Autodesk Inventor part; units mm, degrees
(part 2 of 2)
sketch "スケッチ18" plane through (0, 0, 0) normal (0, 0, 1) x (1, 0, 0)
  line L0 (54.4443, -3) -> (57.4443, -3)
  line L1 (57.4443, -3) -> (57.4443, -6)
  arc A0 (57.4443, -6) -> (59.4443, -6) centre (58.4443, -6) ccw
  line L2 (59.4443, -6) -> (64.4443, -6)
  arc A1 (64.4443, -6) -> (66.4443, -6) centre (65.4443, -6) ccw
  line L3 (66.4443, -6) -> (66.4443, -3)
  line L4 (66.4443, -3) -> (69.4443, -3)
  arc A2 (69.4443, -3) -> (71.4443, -3) centre (70.4443, -3) ccw
  line L5 (71.4443, -3) -> (82.8897, -3)
  arc A3 (82.8897, -3) -> (84.8897, -3) centre (83.8897, -3) ccw
  line L6 (84.8897, -3) -> (87.8897, -3)
  line L7 (87.8897, -3) -> (87.8897, -6)
  arc A4 (87.8897, -6) -> (89.8897, -6) centre (88.8897, -6) ccw
  line L8 (89.8897, -6) -> (94.8897, -6)
  arc A5 (94.8897, -6) -> (96.8897, -6) centre (95.8897, -6) ccw
  line L9 (96.8897, -6) -> (96.8897, -3)
  line L10 (96.8897, -3) -> (99.8897, -3)
  arc A6 (99.8897, -3) -> (101.8897, -3) centre (100.8897, -3) ccw
  line L11 (101.8897, -3) -> (104.885, -3)
  line L12 (104.885, -3) -> (104.885, -31.8586)
  arc A7 (104.885, -31.8586) -> (119.127, -45.896) centre (111.885, -39) ccw
  line L13 (119.127, -45.896) -> (127.6513, -45.7727)
  line L14 (127.6513, -45.7727) -> (121.0577, -50.8686)
  arc A8 (102.2194, -50.4706) -> (121.0577, -50.8686) centre (111.885, -39) ccw
  line L15 (102.2194, -50.4706) -> (49.4443, -6)
  line L16 (49.4443, -6) -> (49.4443, -3)
  line L17 (49.4443, -3) -> (52.4443, -3)
  arc A9 (52.4443, -3) -> (54.4443, -3) centre (53.4443, -3) ccw
  line L18 (99.1203, -14.609) -> (85.9579, -30.2295)
  arc A10 (85.9579, -30.2295) -> (86.0782, -31.6386) centre (86.7226, -30.8739) ccw
  line L19 (86.0782, -31.6386) -> (97.3043, -41.0982)
  arc A11 (97.3043, -41.0982) -> (98.9442, -40.2383) centre (97.9487, -40.3335) ccw
  arc A12 (100.7422, -32.304) -> (98.9442, -40.2383) centre (111.885, -39) ccw
  arc A13 (100.7422, -32.304) -> (100.885, -31.7889) centre (99.885, -31.7889) ccw
  line L20 (100.885, -31.7889) -> (100.885, -15.2534)
  arc A14 (100.885, -15.2534) -> (99.1203, -14.609) centre (99.885, -15.2534) ccw
  line L21 (83.6637, -28.2963) -> (97.8094, -11.5092)
  arc A15 (97.8094, -11.5092) -> (96.8137, -9.8918) centre (97.0447, -10.8648) ccw
  arc A16 (93.4897, -9.2) -> (96.8137, -9.8918) centre (95.8897, -6) ccw
  arc A17 (93.4897, -9.2) -> (92.8897, -9) centre (92.8897, -10) ccw
  line L22 (92.8897, -9) -> (91.8897, -9)
  arc A18 (91.8897, -9) -> (91.2897, -9.2) centre (91.8897, -10) ccw
  arc A19 (85.2178, -7.5865) -> (91.2897, -9.2) centre (88.8897, -6) ccw
  arc A20 (85.2178, -7.5865) -> (84.2178, -6.9865) centre (84.2998, -7.9832) ccw
  arc A21 (81.4897, -6.2) -> (84.2178, -6.9865) centre (83.8897, -3) ccw
  arc A22 (81.4897, -6.2) -> (80.8897, -6) centre (80.8897, -7) ccw
  line L23 (80.8897, -6) -> (73.4443, -6)
  arc A23 (73.4443, -6) -> (72.8443, -6.2) centre (73.4443, -7) ccw
  arc A24 (70.1163, -6.9865) -> (72.8443, -6.2) centre (70.4443, -3) ccw
  arc A25 (70.1163, -6.9865) -> (69.1163, -7.5865) centre (70.0342, -7.9832) ccw
  arc A26 (63.0443, -9.2) -> (69.1163, -7.5865) centre (65.4443, -6) ccw
  arc A27 (63.0443, -9.2) -> (62.4443, -9) centre (62.4443, -10) ccw
  line L24 (62.4443, -9) -> (61.9507, -9)
  arc A28 (61.9507, -9) -> (61.3064, -10.7647) centre (61.9507, -10) ccw
  line L25 (61.3064, -10.7647) -> (82.2546, -28.4167)
  arc A29 (82.2546, -28.4167) -> (83.6637, -28.2963) centre (82.899, -27.652) ccw
  point P0 (0, 0)
  point P1 (0, 0)
  constraints: 60 point on circle, 52 end point, 30 centre point, 12 horizontal, 7 vertical, 123 other
extrude "押し出し22" cut sketch "スケッチ18" against normal blind 4 contours A14 L20 A13 A12 A11 L19 A10 L18 | A29 L25 A28 L24 A27 A26 A25 A24 A23 L23 A22 A21 A20 A19 A18 L22 A17 A16 A15 L21
equation "\"d9\" = d7"
equation "\"d26\" = d7"
